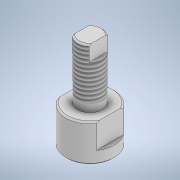
# Autodesk Inventor part: Box Fixing Stud
Saved by Autodesk Inventor 2021 (Build 250183000, 183)
## iProperties
Created: 2020-07-13
Part Number: Box Fixing Stud
Material: Generic
Document SubType Name: Modeling
Designer: jgray
Density: 1 g/cm^3
Appearance: Default
Author: jgray
Autodesk Inventor part; units mm, degrees
ref_plane "YZ Plane" through (0, 0, 0) normal (1, 0, 0) x (0, 1, 0)
ref_plane "XZ Plane" through (0, 0, 0) normal (0, 1, 0) x (-1, 0, 0)
ref_plane "XY Plane" through (0, 0, 0) normal (0, 0, 1) x (1, 0, 0)
sketch "Sketch1" plane through (0, 0, 0) normal (0, 1, 0) x (-1, 0, 0)
  circle A0 centre (0, 0) radius 7.75
  dimension "d0" = 15.5
  constraints: 1 centre point, 1 coincident
  measures "d0" diameter of A0
extrude "Extrusion1" add sketch "Sketch1" along normal blind 12
sketch "Sketch2" plane through (0, 12, 0) normal (0, 1, 0) x (1, 0, 0)
  circle A0 centre (0, 0) radius 7.75 projected
  circle A1 centre (0, 0) radius 7.75 projected
  line L0 (-6.45, -4.2965) -> (-6.45, 4.2965)
  line L1 (6.45, -4.2965) -> (6.45, 4.2965)
  line L2 (0, -12.5996) -> (0, 16.4995) construction
  dimension "d3" = 12.9
  constraints: 6 end point, 4 point on circle, 2 vertical, 1 parallel, 1 point on line, 1 other
  measures "d3" distance between parallel lines of L1 L0
extrude "Extrusion2" cut sketch "Sketch2" against normal blind 8 contours A0 L1 | L0 A0
sketch "Sketch3" plane through (0, 12, 0) normal (0, 1, 0) x (1, 0, 0)
  circle A0 centre (0, 0) radius 4
  dimension "d6" = 8
  constraints: 1 centre point, 1 coincident
  measures "d6" diameter of A0
extrude "Extrusion3" add sketch "Sketch3" along normal blind 19
chamfer "Chamfer1" distance 0.5 angle 45 1 edges at (-4, 31, 0)
thread "Thread1" size "M8x1.25" class "6g" standard "ANSI Metric M Profile" length 16
chamfer "Chamfer2" distance 0.5 angle 45 3 edges at (0, 12, 7.75) (0, 12, -7.75) (7.75, 0, 0)
sketch "Sketch4" plane through (0, 0, 0) normal (0, -1, 0) x (1, 0, 0)
  point P0 (0, 0)
  point P1 (0, 0)
  constraints: 1 coincident
hole "Hole1" at (0, 0, 0) direction (0, 1, 0) diameter 4.917 depth 10 tip angle 118 thread size "M6x1" class "6H" standard "ISO Metric profile"
sketch "Sketch6" plane through (0, 31, 0) normal (0, 1, 0) x (1, 0, 0)
  circle A0 centre (0, 0) radius 4 projected
  line L0 (2.7, -4) -> (-2.7, -4)
  line L1 (-2.7, -4) -> (-2.7, 4)
  line L2 (-2.7, 4) -> (2.7, 4)
  line L3 (2.7, 4) -> (2.7, -4)
  line L4 (2.7, -4) -> (-2.7, 4) construction
  line L5 (-2.7, -4) -> (2.7, 4) construction
  point P0 (-2.7, -2.9513)
  point P1 (-2.7, 2.9513)
  point P2 (2.7, 2.9513)
  point P3 (2.7, -2.9513)
  dimension "d27" = 5.4
  constraints: 12 end point, 2 midpoint, 2 parallel, 1 horizontal, 1 perpendicular, 1 tangent
  measures "d27" distance of L1.end L2.end
extrude "Extrusion5" cut sketch "Sketch6" against normal blind 5 contours A0 L3 | L1 A0
body "Solid1"
